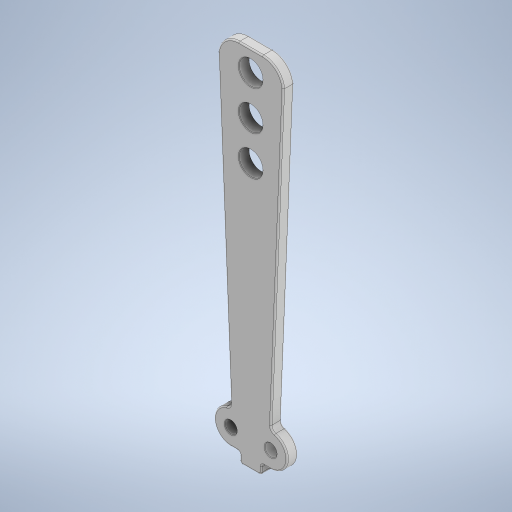
# Autodesk Inventor part: Blade
Saved by Autodesk Inventor 2023.5 (Build 275446000, 446)
## iProperties
Created: 2025-04-03
Part Number: Blade
Material: Generic
Document SubType Name: Modeling
Designer: huy20
Density: 1 g/cm^3
Appearance: Default
Author: huy20
Autodesk Inventor part; units mm, degrees
ref_plane "YZ Plane" through (0, 0, 0) normal (1, 0, 0) x (0, 1, 0)
ref_plane "XZ Plane" through (0, 0, 0) normal (0, 1, 0) x (-1, 0, 0)
ref_plane "XY Plane" through (0, 0, 0) normal (0, 0, 1) x (1, 0, 0)
sketch "Sketch1" plane through (0, 0, 0) normal (0, 0, 1) x (1, 0, 0)
  line L0 (12.495391, 128.318497) -> (7.693564, 14.306579)
  circle A0 centre (-7.620001, 6.211851) radius 2.286
  line L1 (7.619999, 8.497851) -> (7.977609, 8.469707)
  line L2 (7.26239, 3.953996) -> (7.619999, 3.925851)
  circle A1 centre (7.619998, 6.211851) radius 2.286
  arc A2 (-9.197903, 12.362683) -> (-7.620001, -0.138148) centre (-7.620001, 6.211851) ccw
  arc A3 (7.619998, -0.138148) -> (9.198036, 12.362648) centre (7.619998, 6.211851) ccw
  line L3 (-7.693383, 14.306469) -> (-12.492563, 128.318497)
  arc A4 (-4.127501, -2.948149) -> (-3.127501, -3.948149) centre (-3.127501, -2.948149) ccw
  arc A5 (3.127498, -3.948149) -> (4.127498, -2.948149) centre (3.127498, -2.948149) ccw
  line L4 (7.619998, -0.138148) -> (5.127498, -0.138148)
  line L5 (-5.127501, -0.138148) -> (-7.620001, -0.138148)
  arc A6 (-4.127501, -1.138148) -> (-5.127501, -0.138148) centre (-5.127501, -1.138148) ccw
  arc A7 (5.127498, -0.138148) -> (4.127498, -1.138148) centre (5.127498, -1.138148) ccw
  arc A8 (7.696828, 14.384065) -> (9.198036, 12.362648) centre (9.695056, 14.299906) ccw
  arc A9 (-9.197903, 12.362683) -> (-7.696649, 14.384065) centre (-9.69488, 14.299952) ccw
  line L6 (12.495391, 128.318497) -> (12.495391, 135.581738)
  line L7 (12.495391, 135.581738) -> (-12.492563, 135.581738)
  line L8 (-12.492563, 135.581738) -> (-12.492563, 128.318497)
  line L9 (-4.127501, -1.138148) -> (-4.127501, -2.948149)
  line L10 (-3.127501, -3.948149) -> (3.127498, -3.948149)
  line L11 (4.127498, -1.138148) -> (4.127498, -2.948149)
  point P0 (-5.127507, -0.138148)
  point P1 (0.001414, 135.581738)
  point P2 (0, 0)
  dimension "d2" = 15.24
  dimension "d15" = 4.572
  dimension "d16" = 24.98795
  dimension "d17" = 4.82206
  dimension "d74" = 10.16
  dimension "d75" = 3.94815
  dimension "d122" = 2
  constraints: 24 end point, 18 point on circle, 15 tangent, 10 centre point, 6 equal radius, 6 point on line, 4 parallel, 3 coincident, 2 horizontal, 2 vertical, 1 collinear, 1 midpoint
  measures "d2" distance of A1.centre point (-7.62, 6.212)
  measures "d15" diameter of A0
  measures "d16" distance of L6.end L7.end
  measures "d17" angle of L3 L0
  measures "d74" distance from line of L10 A1.centre
  measures "d75" distance from line of L10 point (0, 0)
  measures "d122" radius of A8
sketch "Sketch1 outline for Extrusion1" plane through (0, 0, 0) normal (0, 0, 1) x (1, 0, 0)
  arc A0 (-9.197903, 12.362683) -> (-7.620001, -0.138148) centre (-7.620001, 6.211851) ccw
  arc A1 (-7.696649, 14.384065) -> (-9.197903, 12.362683) centre (-9.69488, 14.299952) cw
  line L0 (-7.620001, -0.138148) -> (-5.127501, -0.138148)
  line L1 (-12.492563, 128.318497) -> (-7.696649, 14.384065)
  arc A2 (-5.127501, -0.138148) -> (-4.127501, -1.138148) centre (-5.127501, -1.138148) cw
  line L2 (-12.492563, 135.581738) -> (-12.492563, 128.318497)
  line L3 (-4.127501, -1.138148) -> (-4.127501, -2.948149)
  line L4 (12.495391, 135.581738) -> (-12.492563, 135.581738)
  arc A3 (-4.127501, -2.948149) -> (-3.127501, -3.948149) centre (-3.127501, -2.948149) ccw
  line L5 (12.495391, 128.318497) -> (12.495391, 135.581738)
  line L6 (-3.127501, -3.948149) -> (3.127498, -3.948149)
  line L7 (7.696828, 14.384065) -> (12.495391, 128.318497)
  arc A4 (3.127498, -3.948149) -> (4.127498, -2.948149) centre (3.127498, -2.948149) ccw
  arc A5 (9.198036, 12.362648) -> (7.696828, 14.384065) centre (9.695056, 14.299906) cw
  line L8 (4.127498, -2.948149) -> (4.127498, -1.138148)
  arc A6 (7.619998, -0.138148) -> (9.198036, 12.362648) centre (7.619998, 6.211851) ccw
  arc A7 (4.127498, -1.138148) -> (5.127498, -0.138148) centre (5.127498, -1.138148) cw
  line L9 (5.127498, -0.138148) -> (7.619998, -0.138148)
  circle A8 centre (-7.620001, 6.211851) radius 2.286
  circle A9 centre (7.619998, 6.211851) radius 2.286
extrude "Extrusion1" add sketch "Sketch1 outline for Extrusion1" along normal mid plane 4.077
fillet "Fillet1" radius 8 2 edges at (12.4954, 135.5817, 0) (-12.4926, 135.5817, 0)
sketch "Sketch2" plane through (0, 0, 2.0385) normal (0, 0, 1) x (1, 0, 0)
  arc A0 (-4.526561, 135.581738) -> (-12.492563, 128.318497) centre (-4.526561, 127.581738) ccw
  line L0 (-12.492563, 128.318497) -> (-7.696649, 14.384065)
  arc A1 (-9.197903, 12.362683) -> (-7.696649, 14.384065) centre (-9.69488, 14.299952) ccw
  arc A2 (-9.197903, 12.362683) -> (-7.620001, -0.138148) centre (-7.620001, 6.211851) ccw
  line L1 (-7.620001, -0.138148) -> (-5.127501, -0.138148)
  arc A3 (-4.127501, -1.138148) -> (-5.127501, -0.138148) centre (-5.127501, -1.138148) ccw
  line L2 (-4.127501, -1.138148) -> (-4.127501, -2.948149)
  arc A4 (-4.127501, -2.948149) -> (-3.127501, -3.948149) centre (-3.127501, -2.948149) ccw
  line L3 (-3.127501, -3.948149) -> (3.127498, -3.948149)
  arc A5 (3.127498, -3.948149) -> (4.127498, -2.948149) centre (3.127498, -2.948149) ccw
  line L4 (4.127498, -2.948149) -> (4.127498, -1.138148)
  arc A6 (5.127498, -0.138148) -> (4.127498, -1.138148) centre (5.127498, -1.138148) ccw
  line L5 (5.127498, -0.138148) -> (7.619998, -0.138148)
  arc A7 (7.619998, -0.138148) -> (9.198036, 12.362648) centre (7.619998, 6.211851) ccw
  arc A8 (7.696828, 14.384065) -> (9.198036, 12.362648) centre (9.695056, 14.299906) ccw
  line L6 (7.696828, 14.384065) -> (12.495391, 128.318497)
  arc A9 (12.495391, 128.318497) -> (4.529389, 135.581738) centre (4.529389, 127.581738) ccw
  line L7 (4.529389, 135.581738) -> (-4.526561, 135.581738)
  circle A10 centre (-7.620001, 6.211851) radius 2.286
  circle A11 centre (7.619998, 6.211851) radius 2.286
  line L8 (-4.526561, 127.581738) -> (4.529389, 127.581738)
  circle A12 centre (0.001414, 127.581738) radius 4.527975
  circle A13 centre (0.001414, 112.581738) radius 4.527975
  circle A14 centre (0.001414, 97.581738) radius 4.527975
  point P0 (0, 0)
  dimension "d114" = 15
  dimension "d115" = 15
  dimension "d118" = 23
  dimension "d119" = 38
  constraints: 2 centre point, 2 end point, 1 horizontal, 1 horizontal alignment, 1 midpoint, 4 other
  measures "d114" distance of A13.centre point (0.001, 127.582)
  measures "d115" distance of A14.centre A13.centre
  measures "d118" distance from line of L7 A13.centre
  measures "d119" distance from line of A14.centre L7
sketch "Sketch2 outline for Extrusion2" plane through (0, 0, 2.0385) normal (0, 0, 1) x (1, 0, 0)
  circle A0 centre (0.001414, 97.581738) radius 4.527975
  circle A1 centre (0.001414, 112.581738) radius 4.527975
  circle A2 centre (0.001414, 127.581738) radius 4.527975
extrude "Extrusion2" cut sketch "Sketch2 outline for Extrusion2" against normal through all
fillet "Fillet3" radius 0.5 36 edges at (9.9195, 133.4933, -2.0385) (-9.9166, 133.4933, -2.0385) (0.0014, 135.5817, -2.0385) (8.0894, 13.1075, -2.0385) (13.92, 5.4166, -2.0385) (6.3737, -0.1381, -2.0385) (4.4204, -0.431, -2.0385) (4.1275, -2.0431, -2.0385) (3.8346, -3.6553, -2.0385) (0, -3.9481, -2.0385) (-3.8346, -3.6553, -2.0385) (-4.1275, -2.0431, -2.0385) (-4.4204, -0.431, -2.0385) (-6.3738, -0.1381, -2.0385) (-13.92, 5.4166, -2.0385) (-8.0893, 13.1075, -2.0385) (-10.0946, 71.3513, -2.0385) (10.0961, 71.3513, -2.0385) (0.0014, 135.5817, 2.0385) (9.9195, 133.4933, 2.0385) (-9.9166, 133.4933, 2.0385) (-8.0893, 13.1075, 2.0385) (-13.92, 5.4166, 2.0385) (-6.3738, -0.1381, 2.0385) (-4.4204, -0.431, 2.0385) (-4.1275, -2.0431, 2.0385) (-3.8346, -3.6553, 2.0385) (0, -3.9481, 2.0385) (3.8346, -3.6553, 2.0385) (4.1275, -2.0431, 2.0385) (4.4204, -0.431, 2.0385) (6.3737, -0.1381, 2.0385) (13.92, 5.4166, 2.0385) (8.0894, 13.1075, 2.0385) (10.0961, 71.3513, 2.0385) (-10.0946, 71.3513, 2.0385)
chamfer "Chamfer1" distance 0.2 angle 45 10 edges at (-9.906, 6.2119, -2.0385) (5.334, 6.2119, -2.0385) (-9.906, 6.2119, 2.0385) (5.334, 6.2119, 2.0385) (-4.5266, 97.5817, 2.0385) (-4.5266, 97.5817, -2.0385) (-4.5266, 112.5817, 2.0385) (-4.5266, 112.5817, -2.0385) (-4.5266, 127.5817, 2.0385) (-4.5266, 127.5817, -2.0385)
body "Solid1"
